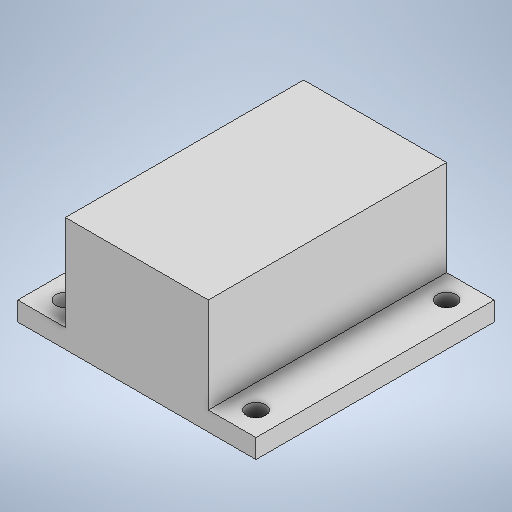
# Autodesk Inventor part: Cube_Stand
Saved by Autodesk Inventor 2026.2 (Build 302298010, 298A)
## iProperties
Created: 2026-05-06
Part Number: Cube_Stand
Material: Generic
Document SubType Name: Modeling
Designer: piete
Density: 1 g/cm^3
Appearance: Default
Author: piete
Autodesk Inventor part; units mm, degrees
ref_plane "YZ Plane" through (0, 0, 0) normal (1, 0, 0) x (0, 1, 0)
ref_plane "XZ Plane" through (0, 0, 0) normal (0, 1, 0) x (-1, 0, 0)
ref_plane "XY Plane" through (0, 0, 0) normal (0, 0, 1) x (1, 0, 0)
sketch "Sketch1" plane through (0, 0, 0) normal (0, 1, 0) x (-1, 0, 0)
  line L0 (15, 25) -> (-15, 25)
  line L1 (-15, 25) -> (-15, -25)
  line L2 (-15, -25) -> (15, -25)
  line L3 (15, -25) -> (15, 25)
  point P0 (0, 0)
  dimension "d0" = 30
  dimension "d1" = 50
  dimension "d2" = 15
  dimension "d3" = 25
  constraints: 8 end point, 2 parallel, 1 horizontal, 1 perpendicular
  measures "d0" distance of L2.end L1.end
  measures "d1" distance of L1.end L0.end
  measures "d2" distance from line of point (0, 0) L3
  measures "d3" distance from line of L0 point (0, 0)
extrude "Extrusion1" add sketch "Sketch1" along normal blind 20
sketch "Sketch2" plane through (0, 0, 0) normal (0, -1, 0) x (1, 0, 0)
  line L0 (-25, 25) -> (25, 25)
  line L1 (25, 25) -> (25, -25)
  line L2 (25, -25) -> (-25, -25)
  line L3 (-25, -25) -> (-25, 25)
  line L4 (-15, 25) -> (15, 25) projected
  line L5 (15, -25) -> (-15, -25) projected
  line L6 (15, 25) -> (15, -25) projected
  line L7 (-15, -25) -> (-15, 25) projected
  circle A0 centre (-20, 20) radius 2
  circle A1 centre (20, 20) radius 2
  circle A2 centre (20, -20) radius 2
  circle A3 centre (-20, -20) radius 2
  point P0 (0, 0)
  dimension "d6" = 0
  dimension "d7" = 0
  dimension "d8" = 10
  dimension "d9" = 10
  dimension "d10" = 4
  dimension "d11" = 4
  dimension "d12" = 4
  dimension "d13" = 4
  dimension "d14" = 5
  dimension "d15" = 5
  dimension "d16" = 5
  dimension "d17" = 5
  dimension "d18" = 5
  dimension "d19" = 5
  dimension "d20" = 5
  dimension "d21" = 5
  constraints: 8 end point, 4 centre point, 2 parallel, 1 horizontal, 1 perpendicular
  measures "d6" distance between parallel lines of L4 L0
  measures "d7" distance between parallel lines of L5 L2
  measures "d8" distance between parallel lines of L6 L1
  measures "d9" distance between parallel lines of L7 L3
  measures "d10" diameter of A0
  measures "d11" diameter of A1
  measures "d12" diameter of A2
  measures "d13" diameter of A3
  measures "d14" distance from line of L0 A0.centre
  measures "d15" distance from line of L3 A0.centre
  measures "d16" distance from line of L1 A1.centre
  measures "d17" distance from line of L0 A1.centre
  measures "d18" distance from line of L1 A2.centre
  measures "d19" distance from line of L2 A2.centre
  measures "d20" distance from line of L3 A3.centre
  measures "d21" distance from line of L2 A3.centre
extrude "Extrusion2" add sketch "Sketch2" along normal blind 4
equation "\"d2\" = 0.5 * d0"
equation "\"d3\" = 0.5 * d1"
body "Solid1"
